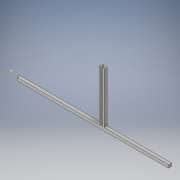
# Autodesk Inventor part: HingeMK3Part2
Saved by Autodesk Inventor 2016 (Build 200138000, 138)
## iProperties
Created: 2017-02-18
Part Number: HingeMK3Part2
Material: Generic
Document SubType Name: Modeling
Designer: RoboticsUser
Density: 1 g/cm^3
Appearance: Default
Mass: 17.0189 g
Surface Area: 122.165 cm^2
Volume: 17.0189 cm^3
Author: RoboticsUser
Autodesk Inventor part; units mm, degrees
ref_plane "YZ Plane" through (0, 0, 0) normal (1, 0, 0) x (0, 1, 0)
ref_plane "XZ Plane" through (0, 0, 0) normal (0, 1, 0) x (-1, 0, 0)
ref_plane "XY Plane" through (0, 0, 0) normal (0, 0, 1) x (1, 0, 0)
sketch "Sketch1" plane through (0, 0, 0) normal (0, 0, 1) x (1, 0, 0)
  line L0 (0, 0) -> (285.75, 0)
  line L1 (285.75, 0) -> (285.75, 6.35)
  line L2 (285.75, 6.35) -> (0, 6.35)
  line L3 (0, 6.35) -> (0, 0)
  dimension "d0" = 285.75
  dimension "d1" = 6.35
  constraints: 8 end point, 2 parallel, 1 horizontal, 1 perpendicular
  measures "d0" distance of L2.end L1.end
  measures "d1" distance of L1.end L0.end
extrude "Extrusion1" add sketch "Sketch1" along normal blind 6.35
sketch "Sketch3" plane through (0, 6.35, 0) normal (0, 1, 0) x (1, 0, 0)
  line L0 (0, -6.35) -> (285.75, -6.35) projected
  line L1 (0, 0) -> (285.75, 0) projected
  line L2 (197.2056, -6.35) -> (200.3806, -6.35)
  line L3 (200.3806, -6.35) -> (200.3806, 0)
  line L4 (200.3806, 0) -> (197.2056, 0)
  line L5 (197.2056, 0) -> (197.2056, -6.35)
  line L6 (192.9892, -6.35) -> (189.8142, -6.35)
  line L7 (189.8142, -6.35) -> (189.8142, 0)
  line L8 (189.8142, 0) -> (192.9892, 0)
  line L9 (192.9892, 0) -> (192.9892, -6.35)
  dimension "d17" = 3.175
  dimension "d18" = 3.175
  constraints: 16 end point, 4 parallel, 4 point on line, 2 horizontal, 2 perpendicular
  measures "d17" distance of L4.end L3.end
  measures "d18" distance of L7.end L8.end
extrude "Extrusion3" add sketch "Sketch3" along normal blind 106.4514 contours L7 L1 L9 L0 | L5 L1 L3 L0
hole "Hole2" at (200.3806, 109.6264, 3.175) direction (-1, 0, 0) diameter 3.175 end through all
sketch "Sketch4" plane through (285.75, 6.35, 6.35) normal (0, 1, 0) x (1, 0, 0)
  point P0 (-285.75, 6.35)
thicken "Thicken1" operation add thickness 26.8986 both sides no extend neighbours yes toward (-1, 0, 0) faces at (285.75, 2.1167, 2.1167)
thicken "Thicken2" operation add thickness 33.4264 both sides no extend neighbours yes toward (1, 0, 0) faces at (0, 4.2333, 2.1167)
thicken "Thicken3" operation add thickness 63.5 both sides no extend neighbours yes toward (1, 0, 0) faces at (258.8514, 2.1167, 2.1167)
thicken "Thicken4" operation add thickness 12.7 both sides no extend neighbours yes toward (1, 0, 0) faces at (322.3514, 2.1167, 2.1167)
thicken "Thicken5" operation add thickness 7.62 both sides no extend neighbours yes toward (-1, 0, 0) faces at (33.4264, 4.2333, 2.1167)
thicken "Thicken6" operation add thickness 7.62 both sides no extend neighbours yes toward (-1, 0, 0) faces at (25.8064, 4.2333, 2.1167)
body "Solid1"
